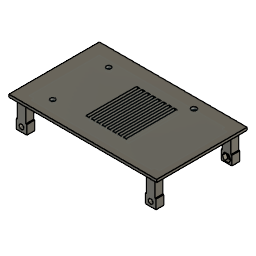
BoTech.StarClock.PowerSupplyTop (Autodesk Fusion 360 design; units mm, degrees)
Autodesk Fusion 360 part; units mm, degrees
note: some values were not read from the file. Set by a fixed rule: which sketch regions a step uses.
sketch "Skizze1" plane through (0, 0, 0) normal (0, 0, 1) x (1, 0, 0)
  line L0 (0, 0) -> (111, 0)
  line L1 (111, 0) -> (111, 68)
  line L2 (0, 68) -> (0, 0)
  line L3 (111, 68) -> (0, 68)
  circle A0 centre (79, 60) radius 2
  line L4 (2, 66) -> (109, 66)
  line L5 (109, 66) -> (109, 2)
  line L6 (109, 2) -> (2, 2)
  line L7 (2, 2) -> (2, 66)
  line L8 (2.5, 66) -> (2.5, 65.5)
  line L9 (2.5, 65.5) -> (2, 65.5)
  line L10 (108.5, 2) -> (108.5, 2.5)
  line L11 (108.5, 2.5) -> (109, 2.5)
  line L12 (2.5, 65.5) -> (108.5, 65.5)
  line L13 (108.5, 65.5) -> (108.5, 2.5)
  line L14 (108.5, 2.5) -> (2.5, 2.5)
  line L15 (2.5, 2.5) -> (2.5, 65.5)
  line L16 (5, 9) -> (35, 9)
  line L17 (35, 9) -> (35, 59)
  line L18 (35, 59) -> (5, 59)
  line L19 (5, 59) -> (5, 9)
  line L20 (20, 9) -> (20, 13)
  circle A1 centre (20, 13) radius 1.75
  line L21 (20, 59) -> (20, 55)
  circle A2 centre (20, 55) radius 1.75
  line L22 (75, 15) -> (73, 15)
  line L23 (73, 15) -> (73, 53)
  line L24 (73, 53) -> (75, 53)
  line L25 (75, 53) -> (75, 15)
  line L26 (71, 53) -> (71, 15)
  line L27 (71, 15) -> (69, 15)
  line L28 (69, 53) -> (71, 53)
  line L29 (69, 15) -> (69, 53)
  line L30 (67, 53) -> (67, 15)
  line L31 (67, 15) -> (65, 15)
  line L32 (65, 53) -> (67, 53)
  line L33 (65, 15) -> (65, 53)
  line L34 (63, 53) -> (63, 15)
  line L35 (63, 15) -> (61, 15)
  line L36 (61, 53) -> (63, 53)
  line L37 (61, 15) -> (61, 53)
  line L38 (59, 53) -> (59, 15)
  line L39 (59, 15) -> (57, 15)
  line L40 (57, 53) -> (59, 53)
  line L41 (57, 15) -> (57, 53)
  line L42 (55, 53) -> (55, 15)
  line L43 (55, 15) -> (53, 15)
  line L44 (53, 53) -> (55, 53)
  line L45 (53, 15) -> (53, 53)
  line L46 (51, 53) -> (51, 15)
  line L47 (51, 15) -> (49, 15)
  line L48 (49, 53) -> (51, 53)
  line L49 (49, 15) -> (49, 53)
  line L50 (47, 53) -> (47, 15)
  line L51 (47, 15) -> (45, 15)
  line L52 (45, 53) -> (47, 53)
  line L53 (45, 15) -> (45, 53)
  line L54 (0, 60) -> (77, 60)
  line L55 (79, 60) -> (79, 66)
  dimension "d9" = 111
  dimension "d10" = 68
  dimension "d13" = 4
  dimension "d30" = 0.5
  dimension "d31" = 0.5
  dimension "d32" = 30
  dimension "d33" = 50
  dimension "d34" = 3.5
  dimension "d35" = 4
  dimension "d36" = 3.5
  dimension "d72" = 2
  dimension "d73" = 38
  dimension "d76" = -28
  dimension "d77" = 0
  dimension "d110" = 77
  dimension "d111" = 6
  constraint horizontal L0
  constraint vertical L1
  constraint horizontal L3
  constraint vertical L2
  constraint coincident L0.start L2.end
  constraint horizontal L4
  constraint vertical L5
  constraint horizontal L6
  constraint vertical L7
  constraint coincident L4 L8.start
  constraint perpendicular L4 L8
  constraint perpendicular L8 L9
  constraint coincident L6 L10.start
  constraint perpendicular L6 L10
  constraint coincident L5 L11.end
  constraint perpendicular L5 L11
  constraint horizontal L12
  constraint vertical L13
  constraint horizontal L14
  constraint vertical L15
  constraint horizontal L16
  constraint vertical L17
  constraint horizontal L18
  constraint vertical L19
  constraint midpoint L16 L20.start
  constraint perpendicular L16 L20
  constraint coincident L20.end A1.centre
  constraint midpoint L18 L21.start
  constraint perpendicular L18 L21
  constraint coincident L21.end A2.centre
  constraint horizontal L22
  constraint vertical L23
  constraint horizontal L24
  constraint vertical L25
  constraint coincident L2 L54.start
  constraint perpendicular L2 L54
  constraint coincident A0.centre L55.start
  constraint perpendicular L4 L55
  measures "d9" distance of L0.start L0.end
  measures "d10" distance of L0.start L2.start
  measures "d13" diameter of A0
  measures "d30" distance of L8.start L8.end
  measures "d31" distance of L10.start L10.end
  measures "d32" distance of L16.start L16.end
  measures "d33" distance of L16.start L18.end
  measures "d34" diameter of A1
  measures "d35" distance of L21.start L21.end
  measures "d36" diameter of A2
  measures "d56" distance of L2.start
  measures "d72" distance of L22.start L22.end
  measures "d73" distance of L22.start L24.end
  measures "d110" distance of L54.start L54.end
  measures "d111" distance of A0.centre L55.end
extrude "Extrusion5" add sketch "Skizze1" along normal blind 2 contours L0 L1 L2 L3 | A0 L12 L15 L54 L55 | A0 L12 L13 L14 L15 L54 L55 | L7 L9 L15 L54 | L6 L7 L10 L14 L15 L54 | L4 L5 L11 L12 L13 L55 | L4 L8 L12 L55 | L4 L7 L8 L9 | L5 L6 L10 L11 | L16 L17 L18 L19
sketch "Skizze3" plane through (0, 53, 0) normal (0, -1, 0) x (1, 0, 0)
  line L0 (73, 0) -> (75, 0)
  line L1 (75, 0) -> (75, 2)
  line L2 (75, 2) -> (73, 2)
  line L3 (73, 2) -> (73, 0)
  line L4 (73, 2) -> (75, 0)
  line L5 (73, 0) -> (71, 2)
  line L6 (71, 2) -> (73, 2)
  line L7 (75, 0) -> (73, 0)
  line L8 (73, 0) -> (71.183, 0)
  line L9 (71.183, 0) -> (71, 2)
  line L10 (71.183, 0) -> (71, 2)
  line L11 (75, 0) -> (75, 2)
  line L12 (73, 2) -> (75, 2)
  line L13 (69, 0) -> (67, 2)
  line L14 (71, 0) -> (71, 2)
  line L15 (69, 2) -> (69, 0)
  line L16 (71, 2) -> (69, 2)
  line L17 (69, 2) -> (71, 2)
  line L18 (71, 0) -> (71, 2)
  line L19 (69, 0) -> (67.183, 0)
  line L20 (69, 2) -> (71, 0)
  line L21 (69, 0) -> (71, 0)
  line L22 (67.183, 0) -> (67, 2)
  line L23 (67, 2) -> (69, 2)
  line L24 (67.183, 0) -> (67, 2)
  line L25 (71, 0) -> (69, 0)
  line L26 (65, 0) -> (63, 2)
  line L27 (67, 0) -> (67, 2)
  line L28 (65, 2) -> (65, 0)
  line L29 (67, 2) -> (65, 2)
  line L30 (65, 2) -> (67, 2)
  line L31 (67, 0) -> (67, 2)
  line L32 (65, 0) -> (63.183, 0)
  line L33 (65, 2) -> (67, 0)
  line L34 (65, 0) -> (67, 0)
  line L35 (63.183, 0) -> (63, 2)
  line L36 (63, 2) -> (65, 2)
  line L37 (63.183, 0) -> (63, 2)
  line L38 (67, 0) -> (65, 0)
  line L39 (61, 0) -> (59, 2)
  line L40 (63, 0) -> (63, 2)
  line L41 (61, 2) -> (61, 0)
  line L42 (63, 2) -> (61, 2)
  line L43 (61, 2) -> (63, 2)
  line L44 (63, 0) -> (63, 2)
  line L45 (61, 0) -> (59.183, 0)
  line L46 (61, 2) -> (63, 0)
  line L47 (61, 0) -> (63, 0)
  line L48 (59.183, 0) -> (59, 2)
  line L49 (59, 2) -> (61, 2)
  line L50 (59.183, 0) -> (59, 2)
  line L51 (63, 0) -> (61, 0)
  line L52 (57, 0) -> (55, 2)
  line L53 (59, 0) -> (59, 2)
  line L54 (57, 2) -> (57, 0)
  line L55 (59, 2) -> (57, 2)
  line L56 (57, 2) -> (59, 2)
  line L57 (59, 0) -> (59, 2)
  line L58 (57, 0) -> (55.183, 0)
  line L59 (57, 2) -> (59, 0)
  line L60 (57, 0) -> (59, 0)
  line L61 (55.183, 0) -> (55, 2)
  line L62 (55, 2) -> (57, 2)
  line L63 (55.183, 0) -> (55, 2)
  line L64 (59, 0) -> (57, 0)
  line L65 (53, 0) -> (51, 2)
  line L66 (55, 0) -> (55, 2)
  line L67 (53, 2) -> (53, 0)
  line L68 (55, 2) -> (53, 2)
  line L69 (53, 2) -> (55, 2)
  line L70 (55, 0) -> (55, 2)
  line L71 (53, 0) -> (51.183, 0)
  line L72 (53, 2) -> (55, 0)
  line L73 (53, 0) -> (55, 0)
  line L74 (51.183, 0) -> (51, 2)
  line L75 (51, 2) -> (53, 2)
  line L76 (51.183, 0) -> (51, 2)
  line L77 (55, 0) -> (53, 0)
  line L78 (49, 0) -> (47, 2)
  line L79 (51, 0) -> (51, 2)
  line L80 (49, 2) -> (49, 0)
  line L81 (51, 2) -> (49, 2)
  line L82 (49, 2) -> (51, 2)
  line L83 (51, 0) -> (51, 2)
  line L84 (49, 0) -> (47.183, 0)
  line L85 (49, 2) -> (51, 0)
  line L86 (49, 0) -> (51, 0)
  line L87 (47.183, 0) -> (47, 2)
  line L88 (47, 2) -> (49, 2)
  line L89 (47.183, 0) -> (47, 2)
  line L90 (51, 0) -> (49, 0)
  line L91 (45, 0) -> (43, 2)
  line L92 (47, 0) -> (47, 2)
  line L93 (45, 2) -> (45, 0)
  line L94 (47, 2) -> (45, 2)
  line L95 (45, 2) -> (47, 2)
  line L96 (47, 0) -> (47, 2)
  line L97 (45, 0) -> (43.183, 0)
  line L98 (45, 2) -> (47, 0)
  line L99 (45, 0) -> (47, 0)
  line L100 (43.183, 0) -> (43, 2)
  line L101 (43, 2) -> (45, 2)
  line L102 (43.183, 0) -> (43, 2)
  line L103 (47, 0) -> (45, 0)
  dimension "d80" = -28
  dimension "d81" = 0
  constraint coincident L2.end L3.start
  constraint coincident L0.end L1.start
  constraint coincident L0.start L3.end
  constraint parallel L4 L5
  constraint perpendicular L3 L6
  constraint perpendicular L3 L8
  constraint coincident L1.end L2.start
extrude "Extrusion8" add sketch "Skizze3" along normal blind 38 contours L92 L94 L95 L96 L98 | L79 L81 L82 L83 L85 | L66 L68 L69 L70 L72 | L53 L55 L56 L57 L59 | L40 L42 L43 L44 L46 | L27 L29 L30 L31 L33 | L14 L16 L17 L18 L20 | L1 L2 L4 L11 L12
extrude "Extrusion9" cut sketch "Skizze3" along normal blind 38 contours L0 L3 L4 L7 | L3 L5 L6 | L15 L20 L21 L25 | L13 L15 L23 | L28 L33 L34 L38 | L26 L28 L36 | L41 L46 L47 L51 | L39 L41 L49 | L54 L59 L60 L64 | L52 L54 L62 | L67 L72 L73 L77 | L65 L67 L75 | L80 L85 L86 L90 | L78 L80 L88 | L93 L98 L99 L103 | L91 L93 L101
sketch "Skizze5" plane through (0, 0, 0) normal (0, 0, 1) x (1, 0, 0)
  line L0 (111, 68) -> (0, 68)
  line L1 (2, 66) -> (109, 66)
  line L2 (108.5, 2) -> (108.5, 2.5)
  line L3 (108.5, 2.5) -> (2.5, 2.5)
  line L4 (0, 0) -> (111, 0)
  line L5 (109, 66) -> (109, 2)
  line L6 (108.5, 2.5) -> (109, 2.5)
  line L7 (2.5, 65.5) -> (108.5, 65.5)
  line L8 (111, 0) -> (111, 68)
  line L9 (2.5, 66) -> (2.5, 65.5)
  line L10 (108.5, 65.5) -> (108.5, 2.5)
  line L11 (109, 2) -> (2, 2)
  line L12 (2, 2) -> (2, 66)
  line L13 (2.5, 65.5) -> (2, 65.5)
  line L14 (0, 68) -> (0, 0)
  line L15 (2.5, 2.5) -> (2.5, 65.5)
  line L16 (108.5, 65.5) -> (104.5, 65.5)
  line L17 (104.5, 65.5) -> (104.5, 61.5)
  line L18 (2.5, 2.5) -> (2.5, 6.5)
  line L19 (2.5, 6.5) -> (6.5, 6.5)
  line L20 (104.5, 61.5) -> (6.5, 61.5)
  line L21 (6.5, 61.5) -> (6.5, 6.5)
  line L22 (6.5, 6.5) -> (104.5, 6.5)
  line L23 (104.5, 6.5) -> (104.5, 61.5)
  circle A0 centre (79, 60) radius 2
  circle A1 centre (79, 60) radius 3
  line L24 (82.5, 61.5) -> (75, 61.5)
  dimension "d138" = 111
  dimension "d139" = 68
  dimension "d141" = 0.5
  dimension "d142" = 0.5
  dimension "d152" = 4
  dimension "d153" = 4
  dimension "d154" = 4
  dimension "d155" = 4
  dimension "d156" = 6
  constraint horizontal L4
  constraint vertical L8
  constraint horizontal L0
  constraint vertical L14
  constraint coincident L4.start L14.end
  constraint horizontal L1
  constraint vertical L5
  constraint horizontal L11
  constraint vertical L12
  constraint coincident L9.start L1
  constraint perpendicular L1 L9
  constraint perpendicular L9 L13
  constraint coincident L2.start L11
  constraint perpendicular L2 L11
  constraint coincident L6.end L5
  constraint perpendicular L5 L6
  constraint horizontal L7
  constraint vertical L10
  constraint horizontal L3
  constraint vertical L15
  constraint coincident L7 L16.end
  constraint perpendicular L7 L17
  constraint coincident L15 L18.end
  constraint perpendicular L15 L19
  constraint horizontal L20
  constraint vertical L21
  constraint horizontal L22
  constraint vertical L23
  constraint concentric A0 A1
  constraint coincident L20 L24.start
  constraint coincident L20 L24.end
  measures "d138" distance of L4.start L4.end
  measures "d139" distance of L0.end L4.start
  measures "d141" distance of L7.start L9.start
  measures "d142" distance of L2.start L2.end
  measures "d152" distance of L7.end L16.end
  measures "d153" distance of L16.end L17.end
  measures "d154" distance of L3.end L18.end
  measures "d155" distance of L18.end L19.end
  measures "d156" diameter of A1
extrude "Extrusion15" add sketch "Skizze5" against normal blind 1.5 contours L7 L15 L17 L19 L20 L21 A1 L24 | L3 L7 L10 L15 L16 L17 L18 L19 L22 L23
sketch "Skizze2" plane through (0, 0, 0) normal (0, -1, 0) x (1, 0, 0)
  line L0 (0, 0) -> (111, 0)
  line L1 (111, 2) -> (0, 2)
  line L2 (0, 2) -> (0, 0)
  circle A0 centre (7, -17) radius 1.75
  line L3 (8.75, -17) -> (10.25, -17)
  line L4 (7.0687, -18.7487) -> (7.0687, -20.2487)
  line L5 (5.25, -17) -> (3.75, -17)
  line L6 (3.75, -17) -> (3.75, -20.25)
  line L7 (3.75, -20.25) -> (7.0687, -20.2487)
  line L8 (7.0687, -20.2487) -> (10.25, -20.25)
  line L9 (10.25, -20.25) -> (10.25, -17)
  line L10 (3.75, -17) -> (3.75, 0)
  line L11 (10.25, -17) -> (10.25, 0)
  line L12 (0, 0) -> (7, 0)
  line L13 (7, 0) -> (7, -17)
  line L14 (55.5, 0) -> (55.5, -30)
  line L15 (0, 0) -> (111, 0)
  line L16 (111, 2) -> (0, 2)
  line L17 (0, 2) -> (0, 0)
  line L18 (5.4123, -14.25) -> (3.8246, -17)
  line L19 (3.8246, -17) -> (5.4123, -19.75)
  line L20 (5.4123, -19.75) -> (8.5877, -19.75)
  line L21 (8.5877, -19.75) -> (10.14, -16.9898)
  line L22 (10.14, -16.9898) -> (8.5877, -14.25)
  line L23 (8.5877, -14.25) -> (5.4123, -14.25)
  line L24 (3, -13.5) -> (11, -13.5)
  line L25 (11, -13.5) -> (11, -20.5)
  line L26 (11, -20.5) -> (3, -20.5)
  line L27 (3, -20.5) -> (3, -13.5)
  line L28 (105.5877, -14.25) -> (107.1754, -17)
  line L29 (100.75, -20.25) -> (100.75, -17)
  line L30 (100, -20.5) -> (108, -20.5)
  line L31 (100.86, -16.9898) -> (102.4123, -14.25)
  line L32 (102.4123, -19.75) -> (100.86, -16.9898)
  line L33 (102.25, -17) -> (100.75, -17)
  line L34 (107.25, -20.25) -> (103.9313, -20.2487)
  line L35 (104, 0) -> (104, -17)
  line L36 (108, -20.5) -> (108, -13.5)
  line L37 (103.9313, -20.2487) -> (100.75, -20.25)
  line L38 (102.4123, -14.25) -> (105.5877, -14.25)
  line L39 (107.1754, -17) -> (105.5877, -19.75)
  circle A1 centre (104, -17) radius 1.75
  line L40 (105.5877, -19.75) -> (102.4123, -19.75)
  line L41 (107.25, -17) -> (107.25, 0)
  line L42 (103.9313, -18.7487) -> (103.9313, -20.2487)
  line L43 (105.75, -17) -> (107.25, -17)
  line L44 (100.75, -17) -> (100.75, 0)
  line L45 (108, -13.5) -> (100, -13.5)
  line L46 (107.25, -17) -> (107.25, -20.25)
  line L47 (100, -13.5) -> (100, -20.5)
  dimension "d46" = 3.5
  dimension "d56" = 1.5
  dimension "d57" = 1.5
  dimension "d58" = 1.5
  dimension "d59" = 7
  dimension "d96" = 8
  dimension "d97" = 7
  constraint coincident A0 L3.start
  constraint coincident A0 L4.start
  constraint coincident A0 L5.start
  constraint perpendicular L5 L6
  constraint coincident L0.start L2.end
  constraint coincident L0 L12.end
  constraint perpendicular L10 L12
  constraint coincident A0.centre L13.end
  constraint midpoint L0 L14.start
  constraint perpendicular L0 L14
  constraint horizontal L24
  constraint vertical L25
  constraint horizontal L26
  constraint vertical L27
  constraint symmetric A0 L14 A1
  constraint symmetric L3.start L14 L33.start
  constraint symmetric L3.end L14 L29.end
  constraint symmetric L4.start L14 L42.start
  constraint symmetric L4.end L14 L34.end
  constraint symmetric L5.start L14 L43.start
  constraint symmetric L5.end L14 L41.start
  constraint symmetric L6.end L14 L34.start
  constraint symmetric L8.end L14 L29.start
  constraint symmetric L10.end L14 L41.end
  constraint symmetric L11.end L14 L44.end
  constraint symmetric L12.end L14 L35.start
  constraint symmetric A0.centre L14 L35.end
  constraint symmetric L14 L19.end L39.end
  constraint symmetric L14 L21.end L31.start
  constraint symmetric L14 L18.end L28.end
  constraint symmetric L14 L22.end L31.end
  constraint symmetric L14 L18.start L28.start
  constraint symmetric L14 L20.end L32.start
  constraint symmetric L14 L24.start L36.end
  constraint symmetric L14 L24.end L45.end
  constraint symmetric L14 L25.end L30.start
  constraint symmetric L14 L26.end L30.end
  measures "d46" diameter of A0
  measures "d56" distance of L3.start L3.end
  measures "d57" distance of L4.start L4.end
  measures "d58" distance of L5.start L5.end
  measures "d59" distance of L0.start L12.end
  measures "d96" distance of L24.start L24.end
  measures "d97" distance of L24.start L26.end
extrude "Extrusion16" add sketch "Skizze2" against normal blind 6 from surface at -2.5 contours L0 L10 L12 L13 L15 L24 | L0 L11 L13 L15 L24 | L5 L10 L13 L18 L23 L24 | L6 L7 L8 L9 L10 L11 L24 L25 L26 L27 | L3 L11 L13 L21 L22 L23 L24 | L4 L5 L6 L7 L19 L20 | A0 L3 L13 L21 L22 L23 | A0 L5 L13 L18 L23 | A0 L4 L5 L19 L20 | L3 L4 L8 L9 L20 L21 | A0 L3 L4 L20 L21 | L0 L15 L35 L44 L45 | L0 L15 L35 L41 L45 | L31 L32 L33 L35 L38 L44 L45 | L29 L30 L34 L36 L37 L41 L44 L45 L46 L47 | L28 L35 L38 L41 L43 L45 | L29 L32 L33 L37 L40 L42 | L28 L35 L38 A1 L43 | L31 L32 L33 L35 L38 A1 | L32 L33 A1 L40 L42 | L34 L39 L40 L42 L43 L46 | L39 A1 L40 L42 L43
extrude "Extrusion17" cut sketch "Skizze2" along normal blind 2.75 from surface at -8.5 contours A0 L3 L13 L21 L22 L23 | A0 L5 L13 L18 L23 | A0 L4 L5 L19 L20 | A0 L3 L4 L20 L21 | L28 L35 L38 A1 L43 | L31 L32 L33 L35 L38 A1 | L32 L33 A1 L40 L42 | L39 A1 L40 L42 L43
extrude "Extrusion18" add sketch "Skizze2" along normal blind 6 from surface at -65.5 contours L0 L15 L35 L44 L45 | L0 L15 L35 L41 L45 | L31 L32 L33 L35 L38 L44 L45 | L29 L30 L34 L36 L37 L41 L44 L45 L46 L47 | L28 L35 L38 L41 L43 L45 | L29 L32 L33 L37 L40 L42 | L28 L35 L38 A1 L43 | L31 L32 L33 L35 L38 A1 | L32 L33 A1 L40 L42 | L34 L39 L40 L42 L43 L46 | L39 A1 L40 L42 L43
extrude "Extrusion19" cut sketch "Skizze2" against normal blind 2.75 from surface at -59.5 contours L28 L35 L38 A1 L43 | L31 L32 L33 L35 L38 A1 | L32 L33 A1 L40 L42 | L39 A1 L40 L42 L43
sketch "Skizze6" plane through (0, 0, 0) normal (0, 0, -1) x (1, 0, 0)
  line L0 (100.75, -61.5) -> (100.75, -59.5)
  line L1 (100.75, -59.5) -> (104.5, -59.5)
  line L2 (104.5, -59.5) -> (104.5, -8.5)
  line L3 (104.5, -8.5) -> (100.75, -8.5)
  line L4 (100.75, -8.5) -> (100.75, -6.5)
  line L5 (100.75, -6.5) -> (10.25, -6.5)
  line L6 (10.25, -6.5) -> (10.25, -8.5)
  line L7 (10.25, -8.5) -> (6.5, -8.5)
  line L8 (6.5, -8.5) -> (6.5, -61.5)
  line L9 (6.5, -61.5) -> (76.4019, -61.5)
  arc A0 (76.4019, -61.5) -> (81.5981, -61.5) centre (79, -60) ccw
  line L10 (81.5981, -61.5) -> (100.75, -61.5)
  line L11 (61, -15) -> (63, -15)
  line L12 (63, -15) -> (63, -53)
  line L13 (63, -53) -> (61, -53)
  line L14 (61, -53) -> (61, -15)
  line L15 (75, -53) -> (73, -53)
  line L16 (73, -53) -> (73, -15)
  line L17 (73, -15) -> (75, -15)
  line L18 (75, -15) -> (75, -53)
  line L19 (49, -15) -> (51, -15)
  line L20 (51, -15) -> (51, -53)
  line L21 (51, -53) -> (49, -53)
  line L22 (49, -53) -> (49, -15)
  line L23 (69, -15) -> (71, -15)
  line L24 (71, -15) -> (71, -53)
  line L25 (71, -53) -> (69, -53)
  line L26 (69, -53) -> (69, -15)
  line L27 (53, -15) -> (55, -15)
  line L28 (55, -15) -> (55, -53)
  line L29 (55, -53) -> (53, -53)
  line L30 (53, -53) -> (53, -15)
  circle A1 centre (79, -60) radius 2
  line L31 (57, -15) -> (59, -15)
  line L32 (59, -15) -> (59, -53)
  line L33 (59, -53) -> (57, -53)
  line L34 (57, -53) -> (57, -15)
  circle A2 centre (20, -13) radius 1.75
  line L35 (65, -15) -> (67, -15)
  line L36 (67, -15) -> (67, -53)
  line L37 (67, -53) -> (65, -53)
  line L38 (65, -53) -> (65, -15)
  circle A3 centre (20, -55) radius 1.75
  line L39 (45, -15) -> (47, -15)
  line L40 (47, -15) -> (47, -53)
  line L41 (47, -53) -> (45, -53)
  line L42 (45, -53) -> (45, -15)
